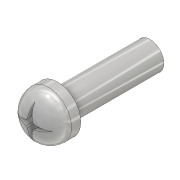
# Autodesk Inventor part: Part7
Saved by Autodesk Inventor 2018 (Build 220112000, 112)
## iProperties
Created: 2020-06-30
Part Number: Part7
Material: Generic
Document SubType Name: Modeling
Designer: IVAN
Density: 1 g/cm^3
Appearance: Aluminum - Polished
Author: IVAN
Autodesk Inventor part; units mm, degrees
ref_plane "YZ Plane" through (0, 0, 0) normal (1, 0, 0) x (0, 1, 0)
ref_plane "XZ Plane" through (0, 0, 0) normal (0, 1, 0) x (-1, 0, 0)
ref_plane "XY Plane" through (0, 0, 0) normal (0, 0, 1) x (1, 0, 0)
sketch "Sketch1" plane through (0, 0, 0) normal (0, 1, 0) x (-1, 0, 0)
  circle A0 centre (0, 0) radius 1.5
  dimension "d0" = 3
  constraints: 1 centre point, 1 coincident
  measures "d0" diameter of A0
extrude "Extrusion1" add sketch "Sketch1" along normal blind 10
sketch "Sketch2" plane through (0, 0, 0) normal (0, -1, 0) x (1, 0, 0)
  circle A0 centre (0, 0) radius 2.5
  dimension "d3" = 5
  constraints: 1 centre point, 1 coincident
  measures "d3" diameter of A0
extrude "Extrusion2" add sketch "Sketch2" along normal blind 3
fillet "Fillet1" radius 2 1 edges at (-2.5, -3, 0)
sketch "Sketch3" plane through (0, -3, 0) normal (0, -1, 0) x (1, 0, 0)
  circle A0 centre (0, 0) radius 0.5 projected
  line L0 (-1.8667, 0) -> (-0.4174, -0.2753)
  circle A1 centre (0, 0) radius 0.5 projected
  line L1 (-1.8667, 0) -> (-0.5, 0)
  dimension "d9" = 0
  constraints: 4 end point, 2 point on circle, 1 horizontal, 1 point on line
  measures "d9" distance from line of point (0, 0) L1
extrude "Extrusion3" cut sketch "Sketch3" against normal blind 2 contours A0 L0 L1
mirror "Mirror1" about plane through (0, 0, 0) normal (0, 0, 1) of "Extrusion3"
pattern_circular "Circular Pattern1" count 4 over 360 about axis through (0, -1, 0) along (0, -1, 0) of "Extrusion3", "Mirror1"
sketch "Sketch4" plane through (0, -3, 0) normal (0, -1, 0) x (1, 0, 0)
  arc A0 (-0.4174, 0.2753) -> (-0.4174, -0.2753) centre (0, 0) ccw projected
  arc A1 (-0.4174, -0.2753) -> (-0.2753, -0.4174) centre (0, 0) ccw projected
  arc A2 (-0.2753, -0.4174) -> (0.2753, -0.4174) centre (0, 0) ccw projected
  arc A3 (0.2753, -0.4174) -> (0.4174, -0.2753) centre (0, 0) ccw projected
  arc A4 (0.4174, -0.2753) -> (0.4174, 0.2753) centre (0, 0) ccw projected
  arc A5 (0.4174, 0.2753) -> (0.2753, 0.4174) centre (0, 0) ccw projected
  arc A6 (0.2753, 0.4174) -> (-0.2753, 0.4174) centre (0, 0) ccw projected
  arc A7 (-0.2753, 0.4174) -> (-0.4174, 0.2753) centre (0, 0) ccw projected
extrude "Extrusion4" cut sketch "Sketch4" against normal up to surface (2 mm away)
body "Solid1"
